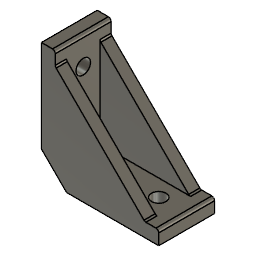
Vslot Corner Joint (Autodesk Fusion 360 design; units mm, degrees)
Autodesk Fusion 360 part; units mm, degrees
sketch "Sketch5" plane through (0, 0, 0) normal (0, 1, 0) x (1, 0, 0)
  line L0 (0, -9) -> (0, -42)
  line L1 (5, -41) -> (5, -37)
  line L2 (4, -42) -> (0, -42)
  line L3 (5, -37) -> (37, -5)
  line L4 (37, -5) -> (41, -5)
  line L5 (42, -4) -> (42, 0)
  arc A0 (4, -42) -> (5, -41) centre (4, -41) ccw
  arc A1 (41, -5) -> (42, -4) centre (41, -4) ccw
  line L6 (0, -9) -> (9, 0)
  line L7 (42, 0) -> (9, 0)
  line L8 (5, -37) -> (5, -11.0711)
  line L9 (5, -11.0711) -> (11.0711, -5)
  line L10 (11.0711, -5) -> (37, -5)
  point P0 (5, -42)
  point P1 (42, -5)
  dimension "d59" = 5
  dimension "d60" = 5
  dimension "d61" = 1
  dimension "d65" = 5
  dimension "d89" = 135
  dimension "d90" = 42
  dimension "d91" = 42
  dimension "d92" = 5
  dimension "d93" = 9
  constraint parallel L0 L1
  constraint perpendicular L0 L2
  constraint horizontal L4
  constraint vertical L5
  constraint coincident P0 L1
  constraint coincident P0 L2
  constraint tangent L1 A0
  constraint tangent L2 A0
  constraint coincident P1 L4
  constraint coincident P1 L5
  constraint tangent L4 A1
  constraint tangent L5 A1
  constraint equal A0 A1
  constraint parallel L1 L8
  constraint parallel L3 L9
  constraint horizontal L10
  constraint horizontal L7
  constraint vertical L0
  constraint horizontal origin L6.end
  constraint vertical origin L0.start
  measures "d59" distance of L5.end P1
  measures "d60" distance of L0.end P0
  measures "d61" radius of A0
  measures "d65" distance of L6 L9
  measures "d89" angle of L6 L7
  measures "d90" distance of L0 L5
  measures "d91" distance of L2 L7
  measures "d92" vertical distance of L1.end L2.start
  measures "d93" distance of origin L6.end
extrude "Extrude14" add sketch "Sketch5" along normal blind 4
extrude "Extrude15" add sketch "Sketch5" along normal blind 20 contours L0 L1 L2 L4 L5 A0 A1 L6 L7 L8 L9 L10
extrude "Extrude16" add sketch "Sketch5" against normal blind 4 from surface at 20
sketch "Sketch6" plane through (0, 0, 5) normal (0, 0, 1) x (-1, 0, 0)
  line L0 (-37, -16) -> (-11.0711, -16)
  line L1 (-11.0711, -16) -> (-11.0711, -4)
  line L2 (-11.0711, -4) -> (-37, -4)
  circle A0 centre (-19, -10) radius 2.5
  circle A1 centre (-32, -10) radius 2.5
  line L3 (-42, 0) -> (-42, -20)
  line L4 (-37, -20) -> (-5, -20)
  line L5 (-37, -4) -> (-37, 0)
  line L6 (-37, 0) -> (-41, 0)
  line L7 (-41, 0) -> (-41, -20)
  line L8 (-41, -20) -> (-37, -20)
  line L9 (-37, -20) -> (-37, -16)
  dimension "d71" = 5
  dimension "d72" = 10
  dimension "d73" = 13
  dimension "d74" = 10
  constraint equal A0 A1
  constraint horizontal A0.centre A1.centre
  measures "d71" diameter of A1
  measures "d72" distance of A1.centre L3
  measures "d73" distance of A0.centre A1.centre
  measures "d74" distance of A1.centre L4
sketch "Sketch7" plane through (5, 0, 0) normal (1, 0, 0) x (0, 1, 0)
  line L0 (20, 41) -> (0, 41)
  line L1 (0, 41) -> (0, 37)
  line L2 (0, 37) -> (4, 37)
  line L3 (4, 37) -> (4, 11.0711)
  line L4 (4, 11.0711) -> (16, 11.0711)
  line L5 (16, 11.0711) -> (16, 37)
  line L6 (16, 37) -> (20, 37)
  line L7 (20, 37) -> (20, 41)
  circle A0 centre (10, 32) radius 2.5
  circle A1 centre (10, 19) radius 2.5
  line L8 (0, 42) -> (20, 42)
  line L9 (0, 37) -> (0, 5)
  dimension "d75" = 5
  dimension "d76" = 10
  dimension "d77" = 13
  dimension "d78" = 10
  constraint equal A0 A1
  constraint vertical A0.centre A1.centre
  measures "d75" diameter of A0
  measures "d76" distance of A0.centre L8
  measures "d77" distance of A0.centre A1.centre
  measures "d78" distance of A0.centre L9
extrude "Extrude17" cut sketch "Sketch7" against normal through all contours A0 | A1
extrude "Extrude18" cut sketch "Sketch6" against normal through all contours A0 | A1
fillet "Fillet5" radius 1 2 edges at (5, 10, 11.0711) (11.0711, 10, 5)
fillet "Fillet6" radius 1 4 edges at (37, 2, 5) (5, 2, 37) (5, 18, 37) (37, 18, 5)
sketch "Sketch8" plane through (0, 0, 0) normal (0, 0, -1) x (1, 0, 0)
  line L0 (42, -20) -> (42, 0)
  line L1 (42, 0) -> (9, 0)
  line L2 (9, 0) -> (9, -20)
  line L3 (9, -20) -> (42, -20)
  line L4 (42, -10) -> (9, -10) construction
  line L5 (42, -6.925) -> (38, -6.925)
  line L6 (38, -6.925) -> (38, -13.075)
  line L7 (38, -13.075) -> (42, -13.075)
  line L8 (42, -13.075) -> (42, -6.925)
  circle A0 centre (19, -10) radius 2.5
  circle A1 centre (32, -10) radius 2.5
  dimension "d87" = 6.15
  dimension "d88" = 4
  constraint midpoint L0 L4.start
  constraint midpoint L2 L4.end
  constraint horizontal L5
  constraint vertical L6
  constraint horizontal L7
  constraint vertical L8
  constraint coincident L0 L5.start
  constraint symmetric L4 L5.end L6.end
  measures "d87" distance of L5.end L6.end
  measures "d88" distance of L6.end L7.end
sketch "Sketch9" plane through (0, 0, 0) normal (-1, 0, 0) x (0, -1, 0)
  circle A0 centre (-10, 32) radius 2.5
  circle A1 centre (-10, 19) radius 2.5
  line L0 (-20, 9) -> (0, 9)
  line L1 (0, 9) -> (0, 42)
  line L2 (0, 42) -> (-20, 42)
  line L3 (-20, 42) -> (-20, 9)
  line L4 (-13.075, 42) -> (-6.925, 42)
  line L5 (-6.925, 42) -> (-6.925, 38)
  line L6 (-6.925, 38) -> (-13.075, 38)
  line L7 (-13.075, 38) -> (-13.075, 42)
  line L8 (-10, 42) -> (-10, 9) construction
  dimension "d98" = 6.15
  dimension "d99" = 4
  constraint horizontal L4
  constraint vertical L5
  constraint horizontal L6
  constraint vertical L7
  constraint coincident L2 L4.start
  constraint midpoint L2 L8.start
  constraint midpoint L0 L8.end
  constraint symmetric L5 L7 L8
  measures "d98" distance of L5.end L6.end
  measures "d99" distance of L4.end L5.end
sketch "Sketch10" plane through (5, 0, 0) normal (1, 0, 0) x (0, 1, 0)
  line L0 (16, 37.4142) -> (20, 37.4142)
  line L1 (20, 37.4142) -> (20, 41)
  line L2 (20, 41) -> (0, 41)
  line L3 (0, 41) -> (0, 37.4142)
  line L4 (0, 37.4142) -> (4, 37.4142)
  line L5 (4, 37.4142) -> (4, 11.4853)
  line L6 (4, 11.4853) -> (16, 11.4853)
  line L7 (16, 11.4853) -> (16, 37.4142)
  circle A0 centre (10, 32) radius 2.5
  circle A1 centre (10, 19) radius 2.5
  circle A2 centre (10, 32) radius 2.6
  circle A3 centre (10, 19) radius 2.6
  dimension "d104" = 5.2
  dimension "d105" = 5.2
  constraint concentric A0 A2
  constraint concentric A1 A3
  measures "d104" diameter of A2
  measures "d105" diameter of A3
extrude "Extrude21" cut sketch "Sketch10" against normal through all contours A0 | A1 | A2 | A3
sketch "Sketch11" plane through (0, 0, 5) normal (0, 0, 1) x (-1, 0, 0)
  circle A0 centre (-32, -10) radius 2.5
  circle A1 centre (-19, -10) radius 2.5
  line L0 (-37.4142, -20) -> (-37.4142, -16)
  line L1 (-37.4142, -16) -> (-11.4853, -16)
  line L2 (-11.4853, -16) -> (-11.4853, -4)
  line L3 (-11.4853, -4) -> (-37.4142, -4)
  line L4 (-37.4142, -4) -> (-37.4142, 0)
  line L5 (-37.4142, 0) -> (-41, 0)
  line L6 (-41, 0) -> (-41, -20)
  line L7 (-41, -20) -> (-37.4142, -20)
  circle A2 centre (-19, -10) radius 2.6
  circle A3 centre (-32, -10) radius 2.6
  dimension "d107" = 5.2
  dimension "d108" = 5.2
  constraint concentric A1 A2
  constraint concentric A0 A3
  measures "d107" diameter of A2
  measures "d108" diameter of A3
extrude "Extrude22" cut sketch "Sketch11" against normal through all contours A0 | A1 | A2 | A3
